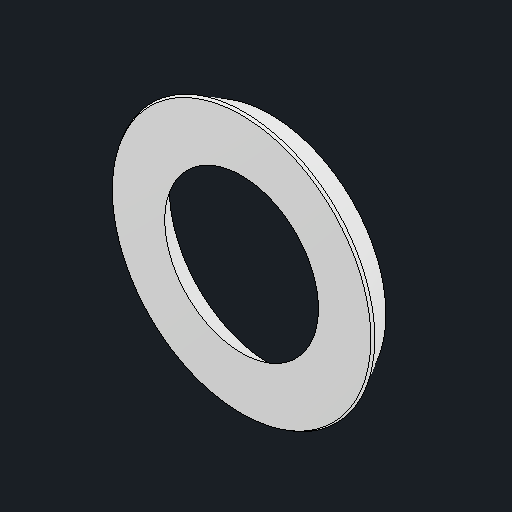
# Autodesk Inventor part: test-external-cone-overhang
Saved by Autodesk Inventor 2026 (Build 300175050, 175E)
## iProperties
Created: 2026-01-09
Part Number: test-external-cone-overhang
Material: ABS Plastic
Document SubType Name: Modeling
Designer: kuzmin
Density: 1.06 g/cm^3
Appearance: Smooth - White
Author: kuzmin
Autodesk Inventor part; units mm, degrees
ref_plane "YZ Plane" through (0, 0, 0) normal (1, 0, 0) x (0, 1, 0)
ref_plane "XZ Plane" through (0, 0, 0) normal (0, 1, 0) x (-1, 0, 0)
ref_plane "XY Plane" through (0, 0, 0) normal (0, 0, 1) x (1, 0, 0)
sketch "Sketch1" plane through (0, 0, 0) normal (0, 1, 0) x (-1, 0, 0)
  line L0 (0, 0) -> (0, 20)
  line L1 (-91.547, 20) -> (-80, 0)
  line L2 (-91.547, 20) -> (-53.218, 20)
  line L3 (-53.218, 20) -> (-70, 0)
  line L4 (-80, 0) -> (-70, 0)
  dimension "d0" = 160
  dimension "d2" = 20
  dimension "d5" = 30
  dimension "d6" = 40
  dimension "d7" = 10
  constraints: 10 end point, 2 horizontal, 2 horizontal alignment, 1 vertical
  measures "d0" diameter of L1.end L0
  measures "d2" distance of L0.start L0.end
  measures "d5" angle of L0 L1
  measures "d6" angle of L0 L3
  measures "d7" distance of L1.end L3.end
revolve "Revolution1" add sketch "Sketch1" angle 360 about axis through (0, 0, 0) along (0, 0, 1)
chamfer "Chamfer1" distance 2 angle 45 1 edges at (-91.547, 0, 20)
equation "\"d5\" = outer"
equation "\"d6\" = inner"
equation "\"outer\" = 30deg"
equation "\"inner\" = 40deg"
body "Solid1"
